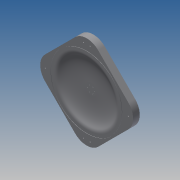
# Autodesk Inventor part: wheel_rim_mold_A
Saved by Autodesk Inventor 2016 (Build 200138000, 138)
## iProperties
Created: 2014-06-11
Part Number: wheel_rim_mold_A
Material: Générique
Document SubType Name: Modeling
Designer: Yann
Density: 1 g/cm^3
Appearance: Par défaut
Mass: 4520.39 g
Surface Area: 4824.92 cm^2
Volume: 4520.39 cm^3
Author: Yann
Autodesk Inventor part; units mm, degrees
ref_plane "YZ Plane" through (0, 0, 0) normal (1, 0, 0) x (0, 1, 0)
ref_plane "XZ Plane" through (0, 0, 0) normal (0, 1, 0) x (-1, 0, 0)
sketch "Esquisse1" plane through (0, 0, 0) normal (0, 1, 0) x (-1, 0, 0)
  circle A0 centre (0, 0) radius 215.2 construction
  line L0 (0, -455.3768) -> (0, 455.3768) projected
  line L1 (-455.3768, 0) -> (455.3768, 0) projected
  line L2 (70.7107, -254.5584) -> (254.5584, -70.7107)
  line L3 (254.5584, 70.7107) -> (70.7107, 254.5584)
  line L4 (-70.7107, 254.5584) -> (-254.5584, 70.7107)
  line L5 (-254.5584, -70.7107) -> (-70.7107, -254.5584)
  line L6 (0, -325.2691) -> (0, 325.2691) construction
  line L7 (325.2691, 0) -> (-325.2691, 0) construction
  circle A1 centre (-20, 253.412) radius 4
  circle A2 centre (11, -19.0526) radius 2.5 projected
  circle A3 centre (-11, -19.0526) radius 2.5 projected
  circle A4 centre (-22, 0) radius 2.5 projected
  circle A5 centre (-11, 19.0526) radius 2.5 projected
  circle A6 centre (11, 19.0526) radius 2.5 projected
  circle A7 centre (22, 0) radius 2.5 projected
  circle A8 centre (0, 0) radius 30 construction
  circle A9 centre (0, 0) radius 13 construction
  arc A10 (-254.5584, 70.7107) -> (-254.5584, -70.7107) centre (-183.8478, 0) ccw
  arc A11 (70.7107, 254.5584) -> (-70.7107, 254.5584) centre (0, 183.8478) ccw
  arc A12 (-70.7107, -254.5584) -> (70.7107, -254.5584) centre (0, -183.8478) ccw
  arc A13 (254.5584, -70.7107) -> (254.5584, 70.7107) centre (183.8478, 0) ccw
  circle A14 centre (20, 253.412) radius 4
  circle A15 centre (-20, -253.412) radius 4
  circle A16 centre (20, -253.412) radius 4
  circle A17 centre (-254.2, 0) radius 4
  circle A18 centre (254.2, 0) radius 4
  point P0 (0, 0)
  dimension "d1" = 460
  dimension "d2" = 8
  dimension "d3" = 35
  dimension "d13" = 100
  dimension "d14" = 20
  dimension "d15" = 35
  constraints: 12 end point, 10 centre point, 9 point on line, 8 point on circle, 8 tangent, 4 equal radius, 4 symmetric about line, 2 midpoint, 2 parallel, 2 perpendicular, 1 horizontal, 4 other
  measures "d1" distance of L6.end L7.start
  measures "d2" diameter of A1
  measures "d13" radius of A10
  measures "d14" distance from line of L6 A1.centre
ref_plane "Plan de construction1" through (-34.1506, 32.18, -34.1506) normal (0, 1, 0) x (0.5, 0, 0.8660254)
extrude "Extrusion1" add sketch "Esquisse1" along normal blind 40.5 contours A12 L5 A10 L1 A17 A4 L0 | L0 L1 A7 A18 A13 L2 A12 | L1 A4 A17 A10 L4 A11 L0 | L0 A11 L3 A13 L1 A18 A7
sketch "Esquisse2" plane through (0, 0, 0) normal (1, 0, 0) x (0, 1, 0)
  line L0 (0, 215.2) -> (0, -215.2) projected
  spline S0 degree 3 poles (0, 200.2) (0, 199.1288) (0.0427, 197.117) (0.1932, 194.8886) (0.4094, 192.844) (0.6322, 191.3431) (0.9669, 189.6041) (1.2775, 188.3098) (1.7156, 186.7818) (2.1051, 185.619) (2.6389, 184.2112) (3.1032, 183.1108) (3.7289, 181.7436) (4.2649, 180.6479) (4.9765, 179.2567) (5.5773, 178.1196) (6.363, 176.6528) (7.017, 175.4374) (7.8605, 173.8529) (8.5535, 172.5284) (9.4365, 170.7907) (10.1537, 169.3309) (11.0581, 167.4098) (11.7859, 165.7925) (12.6956, 163.6626) (13.4217, 161.8692) (14.3225, 159.5092) (15.0362, 157.5244) (15.9156, 154.9177) (16.6075, 152.7301) (17.4542, 149.8647) (18.1158, 147.4666) (18.9197, 144.3355) (19.5431, 141.7234) (20.2945, 138.3249) (20.8724, 135.5001) (21.5631, 131.8402) (22.0894, 128.811) (22.7129, 124.904) (23.1834, 121.6852) (23.7349, 117.5541) (24.1466, 114.1673) (24.6235, 109.8437) (24.9748, 106.3179) (25.3761, 101.842) (25.667, 98.213) (25.9934, 93.6343) (26.2251, 89.945) (26.4792, 85.3215) (26.6546, 81.6221) (26.8408, 77.0209) (26.9641, 73.3685) (27.0885, 68.8656) (27.1653, 65.3246) (27.236, 61.005) (27.2735, 57.6471) (27.3002, 53.6047) (27.307, 50.5086) (27.3014, 46.8466) (27.2875, 44.0985) (27.2632, 40.9295) (27.2402, 38.6236) (27.2152, 36.3262) (27.2005, 34.9709) (27.1891, 33.7716) (27.1821, 32.8731) (27.18, 32.27) (27.18, 32) knots 1 1 1 1 1.041667 1.083333 1.104167 1.145833 1.166667 1.208333 1.229167 1.270833 1.291667 1.333333 1.354167 1.395833 1.416667 1.458333 1.479167 1.520833 1.541667 1.583333 1.604167 1.645833 1.666667 1.708333 1.729167 1.770833 1.791667 1.833333 1.854167 1.895833 1.916667 1.958333 1.979167 2.020833 2.041667 2.083333 2.104167 2.145833 2.166667 2.208333 2.229167 2.270833 2.291667 2.333333 2.354167 2.395833 2.416667 2.458333 2.479167 2.520833 2.541667 2.583333 2.604167 2.645833 2.666667 2.708333 2.729167 2.770833 2.791667 2.833333 2.854167 2.895833 2.916667 2.947917 2.958333 2.979167 3 3 3 3 projected
  line L1 (27.18, 32) -> (27.18, -32) projected
  line L2 (27.18, 0) -> (0, 0)
  line L3 (-10.4655, 0) -> (47.1338, 0) projected
  line L4 (0, 215.2) -> (2, 215.2)
  line L5 (2, 215.2) -> (2, 220.2)
  line L6 (2, 220.2) -> (0, 220.2)
  line L7 (0, 220.2) -> (0, 215.2)
  point P0 (0, 200.1682)
  dimension "d11" = 5
  dimension "d12" = 2
  constraints: 10 end point, 3 parallel, 2 midpoint, 2 perpendicular, 2 other
  measures "d11" distance of L6.end L0.start
  measures "d12" distance of L0.start L4.end
revolve "Révolution1" cut sketch "Esquisse2" angle 360 about axis through (0, -10, 0) along (0, 1, 0)
equation "\"d15\" = d3"
